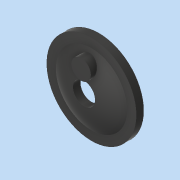
# Autodesk Inventor part: SpurGear
Saved by Autodesk Inventor 2017 (Build 210142000, 142)
## iProperties
Created: 2016-11-06
Part Number: SpurGear
Material: ABS Plastic
Document SubType Name: Modeling
Designer: techn
Density: 1.06 g/cm^3
Appearance: Smooth - Black
Author: techn
Autodesk Inventor part; units mm, degrees
ref_plane "YZ Plane" through (0, 0, 0) normal (1, 0, 0) x (0, 1, 0)
ref_plane "XZ Plane" through (0, 0, 0) normal (0, 1, 0) x (-1, 0, 0)
ref_plane "XY Plane" through (0, 0, 0) normal (0, 0, 1) x (1, 0, 0)
sketch "Sketch1" plane through (0, 0, 0) normal (0, 0, 1) x (1, 0, 0)
  circle A0 centre (0, 0) radius 19.05
  circle A1 centre (0, 0) radius 11.1125
  line L0 (0, 0) -> (0, -12.7)
  circle A2 centre (0, -12.7) radius 4.7625
  circle A3 centre (10.9985, 6.35) radius 4.7625
  circle A4 centre (-10.9985, 6.35) radius 4.7625
  dimension "d0" = 38.1
  dimension "d1" = 22.225
  dimension "d2" = 12.7
  dimension "d3" = 9.525
  dimension "d6" = 360
  constraints: 5 centre point, 3 coincident, 2 end point, 1 vertical, 7 other
  measures "d0" diameter of A0
  measures "d1" diameter of A1
  measures "d2" distance of L0.start L0.end
  measures "d3" diameter of A2
extrude "Extrusion1" add sketch "Sketch1" along normal blind 3.175 contours A0 | A3 A1 | A1 A3 | A2 A1 | A1 L0 A2 | A1 A2 L0 | A4 A1 | A1 A4
sketch "Sketch2" plane through (0, 0, 0) normal (1, 0, 0) x (0, 1, 0)
  line L0 (0, 0) -> (0, 19.3707)
  line L1 (19.05, 3.175) -> (-19.05, 3.175) projected
  line L2 (0, 3.175) -> (15.24, 3.175)
  line L3 (0, 3.175) -> (0, 6.35)
  line L4 (0, 6.35) -> (4.7625, 6.35)
  arc A0 (15.24, 3.175) -> (4.7625, 6.35) centre (1.074, -24.6976) ccw
  line L5 (4.7625, 6.35) -> (4.7625, 3.175)
  dimension "d10" = 15.24
  dimension "d11" = 3.175
  dimension "d12" = 4.7625
  constraints: 10 end point, 3 point on line, 2 point on circle, 2 vertical, 1 centre point, 1 midpoint, 1 perpendicular
  measures "d10" distance of L2.start L2.end
  measures "d11" distance of L2.start L3.end
  measures "d12" distance of L3.end L4.end
revolve "Revolution1" add sketch "Sketch2" angle 360 about axis through (0, 0, 3.175) along (0, 0, 1) contours L5 A0 L1
sketch "Sketch3" plane through (0, 0, 3.175) normal (0, 0, 1) x (1, 0, 0)
  line L0 (0, 0) -> (0, 9.525)
  circle A0 centre (0, 9.525) radius 3.175
  circle A1 centre (0, 9.525) radius 4.1275
  dimension "d14" = 9.525
  dimension "d15" = 6.35
  dimension "d16" = 8.255
  constraints: 2 centre point, 2 coincident, 2 end point, 1 vertical
  measures "d14" distance of L0.start L0.end
  measures "d15" diameter of A0
  measures "d16" diameter of A1
extrude "Extrusion2" add sketch "Sketch3" along normal blind 3.175
sketch "Sketch4" plane through (0, 9.525, 6.35) normal (0, 0, 1) x (1, 0, 0)
  circle A0 centre (0, 0) radius 4.1275 projected
  point P0 (0, -9.525)
extrude "Extrusion3" add sketch "Sketch4" along normal blind 1.27
extrude "Extrusion4" cut sketch "Sketch3" against normal through all contours A0
body "Solid1"
